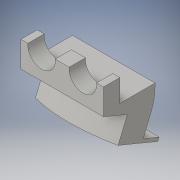
# Autodesk Inventor part: HatSensorMount03FB
Saved by Autodesk Inventor 2016 (Build 200138000, 138)
## iProperties
Created: 2016-12-15
Part Number: HatSensorMount03FB
Material: Generic
Document SubType Name: Modeling
Designer: edozie
Density: 1 g/cm^3
Appearance: Default
Author: edozie
Autodesk Inventor part; units mm, degrees
ref_plane "YZ Plane" through (0, 0, 0) normal (1, 0, 0) x (0, 1, 0)
ref_plane "XZ Plane" through (0, 0, 0) normal (0, 1, 0) x (-1, 0, 0)
ref_plane "XY Plane" through (0, 0, 0) normal (0, 0, 1) x (1, 0, 0)
sketch "Sketch1" plane through (0, 0, 0) normal (0, 0, 1) x (1, 0, 0)
  arc A0 (-19.9373, 1) -> (-4.0627, 1) centre (-12, 0) ccw
  arc A1 (4.0627, 1) -> (19.9373, 1) centre (12, 0) ccw
  line L0 (0, 1) -> (-4.0627, 1)
  line L1 (0, 1) -> (4.0627, 1)
  line L2 (-24, 0) -> (-24, 1)
  line L3 (-19.9373, 1) -> (-24, 1)
  line L4 (24, 0) -> (24, 1)
  line L5 (24, 1) -> (19.9373, 1)
  line L6 (24, 0) -> (24, -12)
  line L7 (24, -12) -> (-24, -12)
  line L8 (-24, -12) -> (-24, 0)
  line L9 (24, 1) -> (24, -12)
  line L10 (24, -12) -> (-24, -12)
  line L11 (-24, -12) -> (-24, 1)
  line L12 (-24, 1) -> (-19.9373, 1)
  line L13 (-4.0627, 1) -> (4.0627, 1)
  line L14 (19.9373, 1) -> (24, 1)
  point P0 (0, 0)
  dimension "d4" = 12
  dimension "d5" = 12
  dimension "d6" = 1
  dimension "d7" = 12
  constraints: 30 end point, 5 parallel, 5 perpendicular, 4 horizontal, 4 point on circle, 2 centre point, 2 vertical
  measures "d4" distance of A0.centre L2.start
  measures "d5" distance of A1.centre L4.start
  measures "d6" distance of L4.start L4.end
  measures "d7" distance of L6.start L6.end
extrude "Extrusion1" add sketch "Sketch1" along normal blind 9.5
sketch "Sketch2" plane through (-24, -12, 0) normal (0, -1, 0) x (1, 0, 0)
  line L0 (0, 9.5) -> (48, 9.5) projected
  line L1 (0, 9.5) -> (48, 9.5)
  line L2 (48, 9.5) -> (48, -20.5)
  line L3 (48, -20.5) -> (0, -20.5)
  line L4 (0, -20.5) -> (0, 9.5)
  point P0 (24, 0)
  dimension "d10" = 30
  constraints: 8 end point, 2 parallel, 1 horizontal, 1 perpendicular
  measures "d10" distance of L1.end L2.end
extrude "Extrusion2" add sketch "Sketch2" along normal blind 2
sketch "Sketch3" plane through (-24, -14, 0) normal (0, -1, 0) x (1, 0, 0)
  line L0 (48, 9.5) -> (0, 9.5) projected
  line L1 (0, 9.5) -> (0, -20.5) projected
  line L2 (0, -20.5) -> (48, -20.5) projected
  line L3 (48, -20.5) -> (48, 9.5) projected
  point P0 (24, 0)
revolve "Revolution1" add sketch "Sketch3" angle 22.5 about axis through (24, -14, 9.5) along (-1, 0, 0)
sketch "Sketch4" plane through (-24, -14, 9.5) normal (0, -0.9238795, 0.3826834) x (1, 0, 0)
  line L0 (48, -27.7164) -> (48, -30) projected
  line L1 (48, -30) -> (0, -30)
  line L2 (0, -30) -> (0, -15)
  line L3 (48, -15) -> (48, -30)
  line L4 (48, -8.0115) -> (48, -26.951) projected
  line L5 (0, -26.951) -> (0, -8.0115) projected
  arc A0 (48, -15) -> (0, -15) centre (24, -70.1) ccw
  point P0 (24, -3.4193)
  constraints: 6 end point, 2 point on circle, 2 point on line, 1 centre point, 1 horizontal, 1 parallel, 1 perpendicular
extrude "Extrusion3" add sketch "Sketch4" along normal blind 12
sketch "Sketch5" plane through (-24, -25.0866, 14.0922) normal (0, -0.9238795, 0.3826834) x (1, 0, 0)
  arc A0 (48, -15) -> (0, -15) centre (24, -70.1) ccw projected
  arc A1 (48, -15) -> (0, -15) centre (24, -70.1) ccw
  line L0 (48, -15) -> (48, -40)
  line L1 (0, -15) -> (0, -40)
  line L2 (0, -40) -> (48, -40)
  point P0 (24, -3.4193)
  dimension "d19" = 25
  dimension "d20" = 25
  constraints: 6 end point, 2 point on circle, 2 vertical, 1 centre point, 1 concentric
  measures "d19" distance of L0.start L0.end
  measures "d20" distance of L1.start L1.end
extrude "Extrusion4" add sketch "Sketch5" along normal blind 2
body "Solid1"
